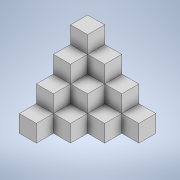
# Autodesk Inventor part: cube_stack
Saved by Autodesk Inventor 2020 (Build 240168000, 168)
## iProperties
Created: 2022-11-14
Part Number: cube_stack
Material: Generic
Document SubType Name: Modeling
Designer: Matthew Ng
Density: 1 g/cm^3
Appearance: Default
Author: Matthew Ng
Autodesk Inventor part; units mm, degrees
ref_plane "YZ Plane" through (0, 0, 0) normal (1, 0, 0) x (0, 1, 0)
ref_plane "XZ Plane" through (0, 0, 0) normal (0, 1, 0) x (-1, 0, 0)
ref_plane "XY Plane" through (0, 0, 0) normal (0, 0, 1) x (1, 0, 0)
sketch "Sketch1" plane through (0, 0, 0) normal (0, 1, 0) x (-1, 0, 0)
  line L0 (0, 0) -> (80, 0)
  line L1 (80, 0) -> (80, -20)
  line L2 (20, -80) -> (0, -80)
  line L3 (0, -80) -> (0, 0)
  line L4 (0, 0) -> (80, 0)
  line L5 (80, 0) -> (80, -20)
  line L6 (80, -20) -> (60, -20)
  line L7 (0, -20) -> (0, 0)
  line L8 (60, -20) -> (60, -40)
  line L9 (60, -40) -> (40, -40)
  line L10 (0, -40) -> (0, -20)
  line L11 (40, -40) -> (40, -60)
  line L12 (40, -60) -> (20, -60)
  line L13 (0, -60) -> (0, -40)
  line L14 (20, -60) -> (20, -80)
  line L15 (20, -80) -> (0, -80)
  line L16 (0, -80) -> (0, -60)
  dimension "d19" = 20
  dimension "d20" = 20
  dimension "d21" = 20
  dimension "d22" = 20
  dimension "d23" = 20
  dimension "d24" = 20
  dimension "d25" = 20
  dimension "d26" = 20
  constraints: 34 end point, 7 parallel, 2 horizontal, 2 perpendicular
  measures "d19" distance between parallel lines of L0 L6
  measures "d20" distance between parallel lines of L9 L6
  measures "d21" distance between parallel lines of L12 L9
  measures "d22" distance from line of L2.start L12
  measures "d23" distance between parallel lines of L8 L1
  measures "d24" distance between parallel lines of L8 L11
  measures "d25" distance between parallel lines of L11 L14
  measures "d26" distance between parallel lines of L3 L14
extrude "Extrusion1" add sketch "Sketch1" along normal blind 20
sketch "Sketch2" plane through (0, 20, 0) normal (0, 1, 0) x (1, 0, 0)
  line L0 (-20, 80) -> (-20, 60) projected
  line L1 (0, 0) -> (0, 80) projected
  line L2 (-20, 60) -> (0, 60)
  line L3 (0, 60) -> (0, 0)
  line L4 (0, 0) -> (-20, 0)
  line L5 (-20, 40) -> (-20, 60)
  line L6 (-40, 60) -> (-40, 40) projected
  line L7 (-40, 40) -> (-20, 40)
  line L8 (-20, 0) -> (-40, 0)
  line L9 (-40, 20) -> (-40, 40)
  line L10 (-60, 20) -> (-80, 20) projected
  line L11 (-60, 20) -> (-40, 20)
  line L12 (-40, 0) -> (-60, 0)
  line L13 (-60, 0) -> (-60, 20)
  dimension "d27" = 20
  constraints: 20 end point, 4 parallel, 3 horizontal, 1 perpendicular
  measures "d27" distance between parallel lines of L13 L9
extrude "Extrusion2" add sketch "Sketch2" along normal blind 20
sketch "Sketch3" plane through (0, 40, 0) normal (0, 1, 0) x (1, 0, 0)
  line L0 (-20, 40) -> (0, 40)
  line L1 (0, 40) -> (0, 0)
  line L2 (0, 0) -> (-20, 0)
  line L3 (-20, 20) -> (-20, 40)
  line L4 (-40, 20) -> (-20, 20)
  line L5 (-20, 0) -> (-40, 0)
  line L6 (-40, 0) -> (-40, 20)
  constraints: 14 end point, 3 parallel, 2 horizontal, 1 perpendicular
extrude "Extrusion3" add sketch "Sketch3" along normal blind 20
sketch "Sketch4" plane through (0, 60, 0) normal (0, 1, 0) x (1, 0, 0)
  line L0 (-20, 20) -> (-20, 40) projected
  line L1 (-20, 20) -> (0, 20)
  line L2 (0, 20) -> (0, 0)
  line L3 (0, 0) -> (-20, 0)
  line L4 (-20, 0) -> (-20, 20)
  constraints: 8 end point, 2 parallel, 1 horizontal, 1 perpendicular
extrude "Extrusion4" add sketch "Sketch4" along normal blind 20
shell "Shell1" thickness 4 removed faces 1 at (-6.6667, 0, -46.6667)
body "Solid1"
